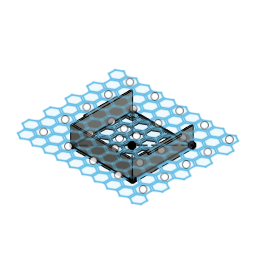
SC846-rear-fan-80mm v2 (Autodesk Fusion 360 design; units mm, degrees)
Autodesk Fusion 360 part; units mm, degrees
sketch "Sketch1" plane through (0, 0, 0) normal (0, 1, 0) x (1, 0, 0)
  line L0 (42.25, -41.5) -> (-42.25, -41.5)
  line L1 (-42.25, -41.5) -> (-42.25, 41.5)
  line L2 (-42.25, 41.5) -> (42.25, 41.5)
  line L3 (42.25, 41.5) -> (42.25, -41.5)
  line L4 (42.25, -41.5) -> (-42.25, 41.5) construction
  line L5 (-42.25, -41.5) -> (42.25, 41.5) construction
  dimension "d1" = 84.5
  dimension "d2" = 83
  constraint horizontal L0
  constraint perpendicular L0 L1
  constraint parallel L0 L2
  constraint parallel L1 L3
  constraint coincident L4 origin
  constraint coincident L5 origin
  measures "d1" distance of L0.start L0.end
  measures "d2" distance of L0.start L2.end
extrude "Extrude1" add sketch "Sketch1" along normal blind 3
sketch "Sketch2" plane through (0, 3, 0) normal (0, 1, 0) x (-1, 0, 0)
  line L0 (-42.25, -41.5) -> (42.25, -41.5)
  line L1 (42.25, -41.5) -> (42.25, 41.5)
  line L2 (42.25, 41.5) -> (-42.25, 41.5)
  line L3 (-42.25, 41.5) -> (-42.25, -41.5)
  line L4 (42.25, 41.5) -> (-42.25, 41.5)
  line L5 (-42.25, 41.5) -> (-42.25, 39.5)
  line L6 (-42.25, 39.5) -> (42.25, 39.5)
  line L7 (42.25, 39.5) -> (42.25, 41.5)
  dimension "d5" = 2
  constraint horizontal L4
  constraint vertical L5
  constraint horizontal L6
  constraint vertical L7
  constraint coincident L3 L5.end
  constraint coincident L1.end L2.start
  measures "d5" distance of L2.end L5.end
extrude "Extrude2" add sketch "Sketch2" along normal blind 24.5 contours L1 L2 L3 L4 L5 L6 L7
sketch "Sketch3" plane through (0, 0, 0) normal (0, 1, 0) x (1, 0, 0)
  line L0 (42.25, 41.5, 3) -> (40.5, 41.5, 3)
  line L1 (40.5, 41.5, 3) -> (40.5, -39.5, 3)
  line L2 (40.5, -39.5, 3) -> (42.25, -39.5, 3)
  line L3 (42.25, -39.5, 3) -> (42.25, 41.5, 3)
  line L4 (-42.25, -39.5, 3) -> (42.25, -39.5, 3)
  point P0 (42.25, 41.5)
  dimension "d8" = 1.75
extrude "Extrude3" add sketch "Sketch3" along normal up to surface (24.5 mm away) contours L0 L1 L2 L3 L4 in plane through (0, 3, 0) normal (0, 1, 0)
sketch "Sketch4" plane through (0, 3, 0) normal (0, 1, 0) x (-1, 0, 0)
  line L0 (-40.5, 39.5) -> (-40.5, -41.5)
  line L1 (-40.5, -41.5) -> (42.25, -41.5)
  line L2 (42.25, -41.5) -> (42.25, 39.5)
  line L3 (42.25, 39.5) -> (-40.5, 39.5)
  line L4 (42.25, 39.5) -> (40.5, 39.5)
  line L5 (40.5, 39.5) -> (40.5, -41.5)
  line L6 (40.5, -41.5) -> (42.25, -41.5)
  line L7 (42.25, -41.5) -> (42.25, 39.5)
  dimension "d11" = 1.75
  constraint horizontal L4
  constraint vertical L5
  constraint horizontal L6
  constraint vertical L7
  constraint coincident L1 L5.end
  constraint coincident L2.end L3.start
  measures "d11" distance of L5.end L1.end
extrude "Extrude4" add sketch "Sketch4" along normal up to surface (24.5 mm away) contours L1 L2 L3 L4 L5 L6 L7
sketch "Sketch5" plane through (0, 3, 0) normal (0, 1, 0) x (-1, 0, 0)
  line L0 (40.5, -41.5) -> (40.5, 39.5)
  line L1 (40.5, 39.5) -> (-40.5, 39.5)
  line L2 (-40.5, 39.5) -> (-40.5, -41.5)
  line L3 (-40.5, -41.5) -> (40.5, -41.5)
  line L4 (-40.5, -41.5) -> (40.5, 39.5) construction
  line L5 (40.5, -41.5) -> (-40.5, 39.5) construction
  constraint coincident L2.end L3.start
  constraint coincident L0.end L1.start
  constraint coincident L0.start L3.end
  constraint coincident L1.end L2.start
sketch "Sketch11" plane through (42.25, 0, 0) normal (1, 0, 0) x (0, 0, -1)
  line L0 (-41.5, 0) -> (41.5, 0)
  line L1 (41.5, 0) -> (41.5, 27.5)
  line L2 (41.5, 27.5) -> (-41.5, 27.5)
  line L3 (-41.5, 27.5) -> (-41.5, 0)
  line L4 (-21.5, 27.5) -> (23.5, 27.5)
  line L5 (23.5, 27.5) -> (23.5, 25)
  line L6 (23.5, 25) -> (-21.5, 25)
  line L7 (-21.5, 25) -> (-21.5, 27.5)
  dimension "d58" = 2.5
  dimension "d59" = 20
  dimension "d60" = 45
  constraint horizontal L4
  constraint vertical L5
  constraint horizontal L6
  constraint vertical L7
  constraint coincident L2 L4.start
  measures "d58" distance of L4.start L6.end
  measures "d59" distance of L3 L7
  measures "d60" distance of L5.end L6.end
extrude "Extrude6" add sketch "Sketch11" along normal blind 2 contours L2 L4 L5 L6 L7
sketch "Sketch12" plane through (-42.25, 0, 0) normal (-1, 0, 0) x (0, 0, 1)
  line L0 (-41.5, 0) -> (41.5, 0)
  line L1 (41.5, 0) -> (41.5, 27.5)
  line L2 (41.5, 27.5) -> (-41.5, 27.5)
  line L3 (-41.5, 27.5) -> (-41.5, 0)
  line L4 (21.5, 27.5) -> (-23.5, 27.5)
  line L5 (-23.5, 27.5) -> (-23.5, 25)
  line L6 (-23.5, 25) -> (21.5, 25)
  line L7 (21.5, 25) -> (21.5, 27.5)
  dimension "d63" = 2.5
  dimension "d64" = 45
  dimension "d65" = 20
  constraint horizontal L4
  constraint vertical L5
  constraint horizontal L6
  constraint vertical L7
  constraint coincident L2 L4.start
  measures "d63" distance of L4.start L6.end
  measures "d64" distance of L5.end L6.end
  measures "d65" distance of L1.end L4.start
extrude "Extrude7" add sketch "Sketch12" along normal blind 2 contours L2 L4 L5 L6 L7
sketch "Sketch13" plane through (0, 3, -1) normal (0, 1, 0) x (-1, 0, 0)
  line L0 (40.5, 40.5) -> (31, 40.5)
  line L1 (31, 40.5) -> (31, 31)
  line L2 (31, 31) -> (40.5, 31)
  line L3 (40.5, 31) -> (40.5, 40.5)
  line L4 (-40.5, -40.5) -> (40.5, 40.5)
  line L5 (40.5, -40.5) -> (31, -40.5)
  line L6 (31, -40.5) -> (31, -31)
  line L7 (31, -31) -> (40.5, -31)
  line L8 (40.5, -31) -> (40.5, -40.5)
  line L9 (40.5, -40.5) -> (-40.5, 40.5)
  line L10 (-40.5, 40.5) -> (-31, 40.5)
  line L11 (-31, 40.5) -> (-31, 31)
  line L12 (-31, 31) -> (-40.5, 31)
  line L13 (-40.5, 31) -> (-40.5, 40.5)
  line L14 (-40.5, -40.5) -> (-31, -40.5)
  line L15 (-31, -40.5) -> (-31, -31)
  line L16 (-31, -31) -> (-40.5, -31)
  line L17 (-40.5, -31) -> (-40.5, -40.5)
  line L18 (40.5, 40.5) -> (-40.5, 40.5)
  line L19 (-40.5, 40.5) -> (-40.5, -40.5)
  line L20 (-40.5, -40.5) -> (40.5, -40.5)
  line L21 (40.5, -40.5) -> (40.5, 40.5)
  line L22 (40.5, 40.5) -> (-40.5, -40.5) construction
  line L23 (-40.5, 40.5) -> (40.5, -40.5) construction
  point P0 (40.5, 40.5)
  point P1 (40.5, -40.5)
  constraint horizontal L0
  constraint vertical L1
  constraint horizontal L2
  constraint vertical L3
  constraint coincident L1.end L4
  constraint coincident P0 L0.start
  constraint horizontal L5
  constraint vertical L6
  constraint horizontal L7
  constraint vertical L8
  constraint coincident L6.end L9
  constraint coincident P1 L5.start
  constraint horizontal L10
  constraint vertical L11
  constraint horizontal L12
  constraint vertical L13
  constraint coincident L9 L11.end
  constraint coincident L9.end L10.start
  constraint horizontal L14
  constraint vertical L15
  constraint horizontal L16
  constraint vertical L17
  constraint coincident L4 L15.end
  constraint coincident L4.start L14.start
  constraint horizontal L18
  constraint perpendicular L18 L19
  constraint parallel L18 L20
  constraint parallel L19 L21
  constraint coincident L22 origin
  constraint coincident L23 origin
extrude "Extrude8" cut sketch "Sketch13" against normal through all contours L1 L4 L9 L11 L18 | L2 L4 L7 L9 L21 | L4 L6 L9 L15 L20 | L4 L9 L12 L16 L19
fillet "Fillet3" radius 4.5 4 edges at (31, 1.5, 30) (-31, 1.5, -32) (-31, 1.5, 30) (31, 1.5, -32)
sketch "Sketch15" plane through (0, 0, -41.5) normal (0, 0, -1) x (-1, 0, 0)
  line L0 (-31, 0) -> (-31, 3)
  line L1 (-31, 3) -> (-40.5, 3)
  line L2 (-40.5, 3) -> (-40.5, 27.5)
  line L3 (-40.5, 27.5) -> (-42.25, 27.5)
  line L4 (-42.25, 27.5) -> (-42.25, 0)
  line L5 (-42.25, 0) -> (-31, 0)
  line L6 (-42.25, 0) -> (42.25, 0)
  line L7 (42.25, 0) -> (42.25, 3)
  line L8 (42.25, 3) -> (-42.25, 3)
  line L9 (-42.25, 3) -> (-42.25, 0)
  line L10 (42.25, 0) -> (42.25, 27.5)
  constraint horizontal L6
  constraint vertical L7
  constraint horizontal L8
  constraint vertical L9
  constraint coincident L7.end L10
  constraint coincident L4.end L5.start
extrude "Extrude9" add sketch "Sketch15" along normal blind 2 contours L0 L1 L4 L5 L6 L8 L9 | L0 L6 L7 L8 L10
sketch "Sketch16" plane through (0, 27.5, 0) normal (0, 1, 0) x (-1, 0, 0)
  line L0 (42.25, 21.5) -> (42.25, 41.5)
  line L1 (42.25, 41.5) -> (-42.25, 41.5)
  line L2 (-42.25, 41.5) -> (-42.25, 21.5)
  line L3 (-42.25, 21.5) -> (-44.25, 21.5)
  line L4 (-44.25, 21.5) -> (-44.25, -23.5)
  line L5 (-44.25, -23.5) -> (-42.25, -23.5)
  line L6 (-42.25, -23.5) -> (-42.25, -41.5)
  line L7 (-42.25, -41.5) -> (-40.5, -41.5)
  line L8 (-40.5, -41.5) -> (-40.5, 39.5)
  line L9 (-40.5, 39.5) -> (40.5, 39.5)
  line L10 (40.5, 39.5) -> (40.5, -41.5)
  line L11 (40.5, -41.5) -> (42.25, -41.5)
  line L12 (42.25, -41.5) -> (42.25, -23.5)
  line L13 (42.25, -23.5) -> (44.25, -23.5)
  line L14 (44.25, -23.5) -> (44.25, 21.5)
  line L15 (44.25, 21.5) -> (42.25, 21.5)
  line L16 (-25.5, 39.5) -> (-20.5, 39.5)
  line L17 (-20.5, 39.5) -> (-20.5, 41.5)
  line L18 (-20.5, 41.5) -> (-25.5, 41.5)
  line L19 (-25.5, 41.5) -> (-25.5, 39.5)
  dimension "d73" = 15
  dimension "d74" = 5
  constraint horizontal L16
  constraint vertical L17
  constraint horizontal L18
  constraint vertical L19
  constraint coincident L1 L17.end
  constraint coincident L9 L16.start
  measures "d73" distance of L8.end L16.start
  measures "d74" distance of L16.start L16.end
extrude "Extrude10" cut sketch "Sketch16" against normal blind 5 contours L1 L9 L16 L17 L18 L19
fillet "Fillet4" radius 1 4 edges at (25.5, 22.5, 40.5) (25.5, 27.5, 40.5) (20.5, 22.5, 40.5) (20.5, 27.5, 40.5)
fillet "Fillet5" radius 1 2 edges at (0, 3, -43.5) (0, 0, -43.5)
sketch "Sketch17" plane through (0, 3, 0) normal (0, 1, 0) x (-1, 0, 0)
  line L0 (-7.5, -4.3301) -> (0, -8.6603)
  line L1 (0, -8.6603) -> (7.5, -4.3301)
  line L2 (7.5, -4.3301) -> (7.5, 4.3301)
  line L3 (7.5, 4.3301) -> (0, 8.6603)
  line L4 (0, 8.6603) -> (-7.5, 4.3301)
  line L5 (-7.5, 4.3301) -> (-7.5, -4.3301)
  line L6 (9.5, -4.3301) -> (17, -8.6603)
  line L7 (17, -8.6603) -> (24.5, -4.3301)
  line L8 (24.5, -4.3301) -> (24.5, 4.3301)
  line L9 (24.5, 4.3301) -> (17, 8.6603)
  line L10 (17, 8.6603) -> (9.5, 4.3301)
  line L11 (9.5, 4.3301) -> (9.5, -4.3301)
  line L12 (1, -19.0526) -> (8.5, -23.3827)
  line L13 (8.5, -23.3827) -> (16, -19.0526)
  line L14 (16, -19.0526) -> (16, -10.3923)
  line L15 (16, -10.3923) -> (8.5, -6.0622)
  line L16 (8.5, -6.0622) -> (1, -10.3923)
  line L17 (1, -10.3923) -> (1, -19.0526)
  line L18 (18, -19.0526) -> (25.5, -23.3827)
  line L19 (25.5, -23.3827) -> (33, -19.0526)
  line L20 (33, -19.0526) -> (33, -10.3923)
  line L21 (33, -10.3923) -> (25.5, -6.0622)
  line L22 (25.5, -6.0622) -> (18, -10.3923)
  line L23 (18, -10.3923) -> (18, -19.0526)
  line L24 (-42.5, -82.3827) -> (-35, -78.0526)
  line L25 (-50, -69.3923) -> (-50, -78.0526)
  line L26 (-52, -69.3923) -> (-59.5, -65.0622)
  line L27 (-60.5, -63.3301) -> (-60.5, -54.6699)
  line L28 (-68, -67.6603) -> (-60.5, -63.3301)
  line L29 (-59.5, -65.0622) -> (-67, -69.3923)
  line L30 (-52, -78.0526) -> (-52, -69.3923)
  line L31 (-59.5, -82.3827) -> (-52, -78.0526)
  line L32 (-67, -78.0526) -> (-59.5, -82.3827)
  line L33 (-67, -69.3923) -> (-67, -78.0526)
  line L34 (-75.5, -63.3301) -> (-68, -67.6603)
  line L35 (-58.5, -63.3301) -> (-51, -67.6603)
  line L36 (-58.5, -54.6699) -> (-58.5, -63.3301)
  line L37 (-60.5, -54.6699) -> (-68, -50.3397)
  line L38 (-68, -50.3397) -> (-75.5, -54.6699)
  line L39 (-75.5, -54.6699) -> (-75.5, -63.3301)
  line L40 (-51, -50.3397) -> (-58.5, -54.6699)
  line L41 (-43.5, -54.6699) -> (-51, -50.3397)
  line L42 (-43.5, -63.3301) -> (-43.5, -54.6699)
  line L43 (-51, -67.6603) -> (-43.5, -63.3301)
  line L44 (-42.5, -65.0622) -> (-50, -69.3923)
  line L45 (-50, -78.0526) -> (-42.5, -82.3827)
  line L46 (-35, -78.0526) -> (-35, -69.3923)
  line L47 (-35, -69.3923) -> (-42.5, -65.0622)
  line L48 (-8.5, -82.3827) -> (-1, -78.0526)
  line L49 (-16, -69.3923) -> (-16, -78.0526)
  line L50 (-18, -69.3923) -> (-25.5, -65.0622)
  line L51 (-26.5, -63.3301) -> (-26.5, -54.6699)
  line L52 (-34, -67.6603) -> (-26.5, -63.3301)
  line L53 (-25.5, -65.0622) -> (-33, -69.3923)
  line L54 (-18, -78.0526) -> (-18, -69.3923)
  line L55 (-25.5, -82.3827) -> (-18, -78.0526)
  line L56 (-33, -78.0526) -> (-25.5, -82.3827)
  line L57 (-33, -69.3923) -> (-33, -78.0526)
  line L58 (-41.5, -63.3301) -> (-34, -67.6603)
  line L59 (-24.5, -63.3301) -> (-17, -67.6603)
  line L60 (-24.5, -54.6699) -> (-24.5, -63.3301)
  line L61 (-26.5, -54.6699) -> (-34, -50.3397)
  line L62 (-34, -50.3397) -> (-41.5, -54.6699)
  line L63 (-41.5, -54.6699) -> (-41.5, -63.3301)
  line L64 (-17, -50.3397) -> (-24.5, -54.6699)
  line L65 (-9.5, -54.6699) -> (-17, -50.3397)
  line L66 (-9.5, -63.3301) -> (-9.5, -54.6699)
  line L67 (-17, -67.6603) -> (-9.5, -63.3301)
  line L68 (-8.5, -65.0622) -> (-16, -69.3923)
  line L69 (-16, -78.0526) -> (-8.5, -82.3827)
  line L70 (-1, -78.0526) -> (-1, -69.3923)
  line L71 (-1, -69.3923) -> (-8.5, -65.0622)
  line L72 (25.5, -82.3827) -> (33, -78.0526)
  line L73 (18, -69.3923) -> (18, -78.0526)
  line L74 (16, -69.3923) -> (8.5, -65.0622)
  line L75 (7.5, -63.3301) -> (7.5, -54.6699)
  line L76 (0, -67.6603) -> (7.5, -63.3301)
  line L77 (8.5, -65.0622) -> (1, -69.3923)
  line L78 (16, -78.0526) -> (16, -69.3923)
  line L79 (8.5, -82.3827) -> (16, -78.0526)
  line L80 (1, -78.0526) -> (8.5, -82.3827)
  line L81 (1, -69.3923) -> (1, -78.0526)
  line L82 (-7.5, -63.3301) -> (0, -67.6603)
  line L83 (9.5, -63.3301) -> (17, -67.6603)
  line L84 (9.5, -54.6699) -> (9.5, -63.3301)
  line L85 (7.5, -54.6699) -> (0, -50.3397)
  line L86 (0, -50.3397) -> (-7.5, -54.6699)
  line L87 (-7.5, -54.6699) -> (-7.5, -63.3301)
  line L88 (17, -50.3397) -> (9.5, -54.6699)
  line L89 (24.5, -54.6699) -> (17, -50.3397)
  line L90 (24.5, -63.3301) -> (24.5, -54.6699)
  line L91 (17, -67.6603) -> (24.5, -63.3301)
  line L92 (25.5, -65.0622) -> (18, -69.3923)
  line L93 (18, -78.0526) -> (25.5, -82.3827)
  line L94 (33, -78.0526) -> (33, -69.3923)
  line L95 (33, -69.3923) -> (25.5, -65.0622)
  line L96 (59.5, -82.3827) -> (67, -78.0526)
  line L97 (52, -69.3923) -> (52, -78.0526)
  line L98 (50, -69.3923) -> (42.5, -65.0622)
  line L99 (41.5, -63.3301) -> (41.5, -54.6699)
  line L100 (34, -67.6603) -> (41.5, -63.3301)
  line L101 (42.5, -65.0622) -> (35, -69.3923)
  line L102 (50, -78.0526) -> (50, -69.3923)
  line L103 (42.5, -82.3827) -> (50, -78.0526)
  line L104 (35, -78.0526) -> (42.5, -82.3827)
  line L105 (35, -69.3923) -> (35, -78.0526)
  line L106 (26.5, -63.3301) -> (34, -67.6603)
  line L107 (43.5, -63.3301) -> (51, -67.6603)
  line L108 (43.5, -54.6699) -> (43.5, -63.3301)
  line L109 (41.5, -54.6699) -> (34, -50.3397)
  line L110 (34, -50.3397) -> (26.5, -54.6699)
  line L111 (26.5, -54.6699) -> (26.5, -63.3301)
  line L112 (51, -50.3397) -> (43.5, -54.6699)
  line L113 (58.5, -54.6699) -> (51, -50.3397)
  line L114 (58.5, -63.3301) -> (58.5, -54.6699)
  line L115 (51, -67.6603) -> (58.5, -63.3301)
  line L116 (59.5, -65.0622) -> (52, -69.3923)
  line L117 (52, -78.0526) -> (59.5, -82.3827)
  line L118 (67, -78.0526) -> (67, -69.3923)
  line L119 (67, -69.3923) -> (59.5, -65.0622)
  line L120 (93.5, -82.3827) -> (101, -78.0526)
  line L121 (86, -69.3923) -> (86, -78.0526)
  line L122 (84, -69.3923) -> (76.5, -65.0622)
  line L123 (75.5, -63.3301) -> (75.5, -54.6699)
  line L124 (68, -67.6603) -> (75.5, -63.3301)
  line L125 (76.5, -65.0622) -> (69, -69.3923)
  line L126 (84, -78.0526) -> (84, -69.3923)
  line L127 (76.5, -82.3827) -> (84, -78.0526)
  line L128 (69, -78.0526) -> (76.5, -82.3827)
  line L129 (69, -69.3923) -> (69, -78.0526)
  line L130 (60.5, -63.3301) -> (68, -67.6603)
  line L131 (77.5, -63.3301) -> (85, -67.6603)
  line L132 (77.5, -54.6699) -> (77.5, -63.3301)
  line L133 (75.5, -54.6699) -> (68, -50.3397)
  line L134 (68, -50.3397) -> (60.5, -54.6699)
  line L135 (60.5, -54.6699) -> (60.5, -63.3301)
  line L136 (85, -50.3397) -> (77.5, -54.6699)
  line L137 (92.5, -54.6699) -> (85, -50.3397)
  line L138 (92.5, -63.3301) -> (92.5, -54.6699)
  line L139 (85, -67.6603) -> (92.5, -63.3301)
  line L140 (93.5, -65.0622) -> (86, -69.3923)
  line L141 (86, -78.0526) -> (93.5, -82.3827)
  line L142 (101, -78.0526) -> (101, -69.3923)
  line L143 (101, -69.3923) -> (93.5, -65.0622)
  line L144 (-42.5, -52.8827) -> (-35, -48.5526)
  line L145 (-50, -39.8923) -> (-50, -48.5526)
  line L146 (-52, -39.8923) -> (-59.5, -35.5622)
  line L147 (-60.5, -33.8301) -> (-60.5, -25.1699)
  line L148 (-68, -38.1603) -> (-60.5, -33.8301)
  line L149 (-59.5, -35.5622) -> (-67, -39.8923)
  line L150 (-52, -48.5526) -> (-52, -39.8923)
  line L151 (-59.5, -52.8827) -> (-52, -48.5526)
  line L152 (-67, -48.5526) -> (-59.5, -52.8827)
  line L153 (-67, -39.8923) -> (-67, -48.5526)
  line L154 (-75.5, -33.8301) -> (-68, -38.1603)
  line L155 (-58.5, -33.8301) -> (-51, -38.1603)
  line L156 (-58.5, -25.1699) -> (-58.5, -33.8301)
  line L157 (-60.5, -25.1699) -> (-68, -20.8397)
  line L158 (-68, -20.8397) -> (-75.5, -25.1699)
  line L159 (-75.5, -25.1699) -> (-75.5, -33.8301)
  line L160 (-51, -20.8397) -> (-58.5, -25.1699)
  line L161 (-43.5, -25.1699) -> (-51, -20.8397)
  line L162 (-43.5, -33.8301) -> (-43.5, -25.1699)
  line L163 (-51, -38.1603) -> (-43.5, -33.8301)
  line L164 (-42.5, -35.5622) -> (-50, -39.8923)
  line L165 (-50, -48.5526) -> (-42.5, -52.8827)
  line L166 (-35, -48.5526) -> (-35, -39.8923)
  line L167 (-35, -39.8923) -> (-42.5, -35.5622)
  line L168 (-8.5, -52.8827) -> (-1, -48.5526)
  line L169 (-16, -39.8923) -> (-16, -48.5526)
  line L170 (-18, -39.8923) -> (-25.5, -35.5622)
  line L171 (-26.5, -33.8301) -> (-26.5, -25.1699)
  line L172 (-34, -38.1603) -> (-26.5, -33.8301)
  line L173 (-25.5, -35.5622) -> (-33, -39.8923)
  line L174 (-18, -48.5526) -> (-18, -39.8923)
  line L175 (-25.5, -52.8827) -> (-18, -48.5526)
  line L176 (-33, -48.5526) -> (-25.5, -52.8827)
  line L177 (-33, -39.8923) -> (-33, -48.5526)
  line L178 (-41.5, -33.8301) -> (-34, -38.1603)
  line L179 (-24.5, -33.8301) -> (-17, -38.1603)
  line L180 (-24.5, -25.1699) -> (-24.5, -33.8301)
  line L181 (-26.5, -25.1699) -> (-34, -20.8397)
  line L182 (-34, -20.8397) -> (-41.5, -25.1699)
  line L183 (-41.5, -25.1699) -> (-41.5, -33.8301)
  line L184 (-17, -20.8397) -> (-24.5, -25.1699)
  line L185 (-9.5, -25.1699) -> (-17, -20.8397)
  line L186 (-9.5, -33.8301) -> (-9.5, -25.1699)
  line L187 (-17, -38.1603) -> (-9.5, -33.8301)
  line L188 (-8.5, -35.5622) -> (-16, -39.8923)
  line L189 (-16, -48.5526) -> (-8.5, -52.8827)
  line L190 (-1, -48.5526) -> (-1, -39.8923)
  line L191 (-1, -39.8923) -> (-8.5, -35.5622)
  line L192 (25.5, -52.8827) -> (33, -48.5526)
  line L193 (18, -39.8923) -> (18, -48.5526)
  line L194 (16, -39.8923) -> (8.5, -35.5622)
  line L195 (7.5, -33.8301) -> (7.5, -25.1699)
  line L196 (0, -38.1603) -> (7.5, -33.8301)
  line L197 (8.5, -35.5622) -> (1, -39.8923)
  line L198 (16, -48.5526) -> (16, -39.8923)
  line L199 (8.5, -52.8827) -> (16, -48.5526)
  line L200 (1, -48.5526) -> (8.5, -52.8827)
  line L201 (1, -39.8923) -> (1, -48.5526)
  line L202 (-7.5, -33.8301) -> (0, -38.1603)
  line L203 (9.5, -33.8301) -> (17, -38.1603)
  line L204 (9.5, -25.1699) -> (9.5, -33.8301)
  line L205 (7.5, -25.1699) -> (0, -20.8397)
  line L206 (0, -20.8397) -> (-7.5, -25.1699)
  line L207 (-7.5, -25.1699) -> (-7.5, -33.8301)
  line L208 (17, -20.8397) -> (9.5, -25.1699)
  line L209 (24.5, -25.1699) -> (17, -20.8397)
  line L210 (24.5, -33.8301) -> (24.5, -25.1699)
  line L211 (17, -38.1603) -> (24.5, -33.8301)
  line L212 (25.5, -35.5622) -> (18, -39.8923)
  line L213 (18, -48.5526) -> (25.5, -52.8827)
  line L214 (33, -48.5526) -> (33, -39.8923)
  line L215 (33, -39.8923) -> (25.5, -35.5622)
  line L216 (59.5, -52.8827) -> (67, -48.5526)
  line L217 (52, -39.8923) -> (52, -48.5526)
  line L218 (50, -39.8923) -> (42.5, -35.5622)
  line L219 (41.5, -33.8301) -> (41.5, -25.1699)
  line L220 (34, -38.1603) -> (41.5, -33.8301)
  line L221 (42.5, -35.5622) -> (35, -39.8923)
  line L222 (50, -48.5526) -> (50, -39.8923)
  line L223 (42.5, -52.8827) -> (50, -48.5526)
  line L224 (35, -48.5526) -> (42.5, -52.8827)
  line L225 (35, -39.8923) -> (35, -48.5526)
  line L226 (26.5, -33.8301) -> (34, -38.1603)
  line L227 (43.5, -33.8301) -> (51, -38.1603)
  line L228 (43.5, -25.1699) -> (43.5, -33.8301)
  line L229 (41.5, -25.1699) -> (34, -20.8397)
  line L230 (34, -20.8397) -> (26.5, -25.1699)
  line L231 (26.5, -25.1699) -> (26.5, -33.8301)
  line L232 (51, -20.8397) -> (43.5, -25.1699)
  line L233 (58.5, -25.1699) -> (51, -20.8397)
  line L234 (58.5, -33.8301) -> (58.5, -25.1699)
  line L235 (51, -38.1603) -> (58.5, -33.8301)
  line L236 (59.5, -35.5622) -> (52, -39.8923)
  line L237 (52, -48.5526) -> (59.5, -52.8827)
  line L238 (67, -48.5526) -> (67, -39.8923)
  line L239 (67, -39.8923) -> (59.5, -35.5622)
  line L240 (93.5, -52.8827) -> (101, -48.5526)
  line L241 (86, -39.8923) -> (86, -48.5526)
  line L242 (84, -39.8923) -> (76.5, -35.5622)
  line L243 (75.5, -33.8301) -> (75.5, -25.1699)
  line L244 (68, -38.1603) -> (75.5, -33.8301)
  line L245 (76.5, -35.5622) -> (69, -39.8923)
  line L246 (84, -48.5526) -> (84, -39.8923)
  line L247 (76.5, -52.8827) -> (84, -48.5526)
  line L248 (69, -48.5526) -> (76.5, -52.8827)
  line L249 (69, -39.8923) -> (69, -48.5526)
  line L250 (60.5, -33.8301) -> (68, -38.1603)
  line L251 (77.5, -33.8301) -> (85, -38.1603)
  line L252 (77.5, -25.1699) -> (77.5, -33.8301)
  line L253 (75.5, -25.1699) -> (68, -20.8397)
  line L254 (68, -20.8397) -> (60.5, -25.1699)
  line L255 (60.5, -25.1699) -> (60.5, -33.8301)
  line L256 (85, -20.8397) -> (77.5, -25.1699)
  line L257 (92.5, -25.1699) -> (85, -20.8397)
  line L258 (92.5, -33.8301) -> (92.5, -25.1699)
  line L259 (85, -38.1603) -> (92.5, -33.8301)
  line L260 (93.5, -35.5622) -> (86, -39.8923)
  line L261 (86, -48.5526) -> (93.5, -52.8827)
  line L262 (101, -48.5526) -> (101, -39.8923)
  line L263 (101, -39.8923) -> (93.5, -35.5622)
  line L264 (-42.5, -23.3827) -> (-35, -19.0526)
  line L265 (-50, -10.3923) -> (-50, -19.0526)
  line L266 (-52, -10.3923) -> (-59.5, -6.0622)
  line L267 (-60.5, -4.3301) -> (-60.5, 4.3301)
  line L268 (-68, -8.6603) -> (-60.5, -4.3301)
  line L269 (-59.5, -6.0622) -> (-67, -10.3923)
  line L270 (-52, -19.0526) -> (-52, -10.3923)
  line L271 (-59.5, -23.3827) -> (-52, -19.0526)
  line L272 (-67, -19.0526) -> (-59.5, -23.3827)
  line L273 (-67, -10.3923) -> (-67, -19.0526)
  line L274 (-75.5, -4.3301) -> (-68, -8.6603)
  line L275 (-58.5, -4.3301) -> (-51, -8.6603)
  line L276 (-58.5, 4.3301) -> (-58.5, -4.3301)
  line L277 (-60.5, 4.3301) -> (-68, 8.6603)
  line L278 (-68, 8.6603) -> (-75.5, 4.3301)
  line L279 (-75.5, 4.3301) -> (-75.5, -4.3301)
  line L280 (-51, 8.6603) -> (-58.5, 4.3301)
  line L281 (-43.5, 4.3301) -> (-51, 8.6603)
  line L282 (-43.5, -4.3301) -> (-43.5, 4.3301)
  line L283 (-51, -8.6603) -> (-43.5, -4.3301)
  line L284 (-42.5, -6.0622) -> (-50, -10.3923)
  line L285 (-50, -19.0526) -> (-42.5, -23.3827)
  line L286 (-35, -19.0526) -> (-35, -10.3923)
  line L287 (-35, -10.3923) -> (-42.5, -6.0622)
  line L288 (-8.5, -23.3827) -> (-1, -19.0526)
  line L289 (-16, -10.3923) -> (-16, -19.0526)
  line L290 (-18, -10.3923) -> (-25.5, -6.0622)
  line L291 (-26.5, -4.3301) -> (-26.5, 4.3301)
  line L292 (-34, -8.6603) -> (-26.5, -4.3301)
  line L293 (-25.5, -6.0622) -> (-33, -10.3923)
  line L294 (-18, -19.0526) -> (-18, -10.3923)
  line L295 (-25.5, -23.3827) -> (-18, -19.0526)
  line L296 (-33, -19.0526) -> (-25.5, -23.3827)
  line L297 (-33, -10.3923) -> (-33, -19.0526)
  line L298 (-41.5, -4.3301) -> (-34, -8.6603)
  line L299 (-24.5, -4.3301) -> (-17, -8.6603)
  line L300 (-24.5, 4.3301) -> (-24.5, -4.3301)
  line L301 (-26.5, 4.3301) -> (-34, 8.6603)
  line L302 (-34, 8.6603) -> (-41.5, 4.3301)
  line L303 (-41.5, 4.3301) -> (-41.5, -4.3301)
  line L304 (-17, 8.6603) -> (-24.5, 4.3301)
  line L305 (-9.5, 4.3301) -> (-17, 8.6603)
  line L306 (-9.5, -4.3301) -> (-9.5, 4.3301)
  line L307 (-17, -8.6603) -> (-9.5, -4.3301)
  line L308 (-8.5, -6.0622) -> (-16, -10.3923)
  line L309 (-16, -19.0526) -> (-8.5, -23.3827)
  line L310 (-1, -19.0526) -> (-1, -10.3923)
  line L311 (-1, -10.3923) -> (-8.5, -6.0622)
  line L312 (59.5, -23.3827) -> (67, -19.0526)
  line L313 (52, -10.3923) -> (52, -19.0526)
  line L314 (50, -10.3923) -> (42.5, -6.0622)
  line L315 (41.5, -4.3301) -> (41.5, 4.3301)
  line L316 (34, -8.6603) -> (41.5, -4.3301)
  line L317 (42.5, -6.0622) -> (35, -10.3923)
  line L318 (50, -19.0526) -> (50, -10.3923)
  line L319 (42.5, -23.3827) -> (50, -19.0526)
  line L320 (35, -19.0526) -> (42.5, -23.3827)
  line L321 (35, -10.3923) -> (35, -19.0526)
  line L322 (26.5, -4.3301) -> (34, -8.6603)
  line L323 (43.5, -4.3301) -> (51, -8.6603)
  line L324 (43.5, 4.3301) -> (43.5, -4.3301)
  line L325 (41.5, 4.3301) -> (34, 8.6603)
  line L326 (34, 8.6603) -> (26.5, 4.3301)
  line L327 (26.5, 4.3301) -> (26.5, -4.3301)
  line L328 (51, 8.6603) -> (43.5, 4.3301)
  line L329 (58.5, 4.3301) -> (51, 8.6603)
  line L330 (58.5, -4.3301) -> (58.5, 4.3301)
  line L331 (51, -8.6603) -> (58.5, -4.3301)
  line L332 (59.5, -6.0622) -> (52, -10.3923)
  line L333 (52, -19.0526) -> (59.5, -23.3827)
  line L334 (67, -19.0526) -> (67, -10.3923)
  line L335 (67, -10.3923) -> (59.5, -6.0622)
  line L336 (93.5, -23.3827) -> (101, -19.0526)
  line L337 (86, -10.3923) -> (86, -19.0526)
  line L338 (84, -10.3923) -> (76.5, -6.0622)
  line L339 (75.5, -4.3301) -> (75.5, 4.3301)
  line L340 (68, -8.6603) -> (75.5, -4.3301)
  line L341 (76.5, -6.0622) -> (69, -10.3923)
  line L342 (84, -19.0526) -> (84, -10.3923)
  line L343 (76.5, -23.3827) -> (84, -19.0526)
  line L344 (69, -19.0526) -> (76.5, -23.3827)
  line L345 (69, -10.3923) -> (69, -19.0526)
  line L346 (60.5, -4.3301) -> (68, -8.6603)
  line L347 (77.5, -4.3301) -> (85, -8.6603)
  line L348 (77.5, 4.3301) -> (77.5, -4.3301)
  line L349 (75.5, 4.3301) -> (68, 8.6603)
  line L350 (68, 8.6603) -> (60.5, 4.3301)
  line L351 (60.5, 4.3301) -> (60.5, -4.3301)
  line L352 (85, 8.6603) -> (77.5, 4.3301)
  line L353 (92.5, 4.3301) -> (85, 8.6603)
  line L354 (92.5, -4.3301) -> (92.5, 4.3301)
  line L355 (85, -8.6603) -> (92.5, -4.3301)
  line L356 (93.5, -6.0622) -> (86, -10.3923)
  line L357 (86, -19.0526) -> (93.5, -23.3827)
  line L358 (101, -19.0526) -> (101, -10.3923)
  line L359 (101, -10.3923) -> (93.5, -6.0622)
  line L360 (-42.5, 6.1173) -> (-35, 10.4474)
  line L361 (-50, 19.1077) -> (-50, 10.4474)
  line L362 (-52, 19.1077) -> (-59.5, 23.4378)
  line L363 (-60.5, 25.1699) -> (-60.5, 33.8301)
  line L364 (-68, 20.8397) -> (-60.5, 25.1699)
  line L365 (-59.5, 23.4378) -> (-67, 19.1077)
  line L366 (-52, 10.4474) -> (-52, 19.1077)
  line L367 (-59.5, 6.1173) -> (-52, 10.4474)
  line L368 (-67, 10.4474) -> (-59.5, 6.1173)
  line L369 (-67, 19.1077) -> (-67, 10.4474)
  line L370 (-75.5, 25.1699) -> (-68, 20.8397)
  line L371 (-58.5, 25.1699) -> (-51, 20.8397)
  line L372 (-58.5, 33.8301) -> (-58.5, 25.1699)
  line L373 (-60.5, 33.8301) -> (-68, 38.1603)
  line L374 (-68, 38.1603) -> (-75.5, 33.8301)
  line L375 (-75.5, 33.8301) -> (-75.5, 25.1699)
  line L376 (-51, 38.1603) -> (-58.5, 33.8301)
  line L377 (-43.5, 33.8301) -> (-51, 38.1603)
  line L378 (-43.5, 25.1699) -> (-43.5, 33.8301)
  line L379 (-51, 20.8397) -> (-43.5, 25.1699)
  line L380 (-42.5, 23.4378) -> (-50, 19.1077)
  line L381 (-50, 10.4474) -> (-42.5, 6.1173)
  line L382 (-35, 10.4474) -> (-35, 19.1077)
  line L383 (-35, 19.1077) -> (-42.5, 23.4378)
  line L384 (-8.5, 6.1173) -> (-1, 10.4474)
  line L385 (-16, 19.1077) -> (-16, 10.4474)
  line L386 (-18, 19.1077) -> (-25.5, 23.4378)
  line L387 (-26.5, 25.1699) -> (-26.5, 33.8301)
  line L388 (-34, 20.8397) -> (-26.5, 25.1699)
  line L389 (-25.5, 23.4378) -> (-33, 19.1077)
  line L390 (-18, 10.4474) -> (-18, 19.1077)
  line L391 (-25.5, 6.1173) -> (-18, 10.4474)
  line L392 (-33, 10.4474) -> (-25.5, 6.1173)
  line L393 (-33, 19.1077) -> (-33, 10.4474)
  line L394 (-41.5, 25.1699) -> (-34, 20.8397)
  line L395 (-24.5, 25.1699) -> (-17, 20.8397)
  line L396 (-24.5, 33.8301) -> (-24.5, 25.1699)
  line L397 (-26.5, 33.8301) -> (-34, 38.1603)
  line L398 (-34, 38.1603) -> (-41.5, 33.8301)
  line L399 (-41.5, 33.8301) -> (-41.5, 25.1699)
  line L400 (-17, 38.1603) -> (-24.5, 33.8301)
  line L401 (-9.5, 33.8301) -> (-17, 38.1603)
  line L402 (-9.5, 25.1699) -> (-9.5, 33.8301)
  line L403 (-17, 20.8397) -> (-9.5, 25.1699)
  line L404 (-8.5, 23.4378) -> (-16, 19.1077)
  line L405 (-16, 10.4474) -> (-8.5, 6.1173)
  line L406 (-1, 10.4474) -> (-1, 19.1077)
  line L407 (-1, 19.1077) -> (-8.5, 23.4378)
  line L408 (25.5, 6.1173) -> (33, 10.4474)
  line L409 (18, 19.1077) -> (18, 10.4474)
  line L410 (16, 19.1077) -> (8.5, 23.4378)
  line L411 (7.5, 25.1699) -> (7.5, 33.8301)
  line L412 (0, 20.8397) -> (7.5, 25.1699)
  line L413 (8.5, 23.4378) -> (1, 19.1077)
  line L414 (16, 10.4474) -> (16, 19.1077)
  line L415 (8.5, 6.1173) -> (16, 10.4474)
  line L416 (1, 10.4474) -> (8.5, 6.1173)
  line L417 (1, 19.1077) -> (1, 10.4474)
  line L418 (-7.5, 25.1699) -> (0, 20.8397)
  line L419 (9.5, 25.1699) -> (17, 20.8397)
  line L420 (9.5, 33.8301) -> (9.5, 25.1699)
  line L421 (7.5, 33.8301) -> (0, 38.1603)
  line L422 (0, 38.1603) -> (-7.5, 33.8301)
  line L423 (-7.5, 33.8301) -> (-7.5, 25.1699)
  line L424 (17, 38.1603) -> (9.5, 33.8301)
  line L425 (24.5, 33.8301) -> (17, 38.1603)
  line L426 (24.5, 25.1699) -> (24.5, 33.8301)
  line L427 (17, 20.8397) -> (24.5, 25.1699)
  line L428 (25.5, 23.4378) -> (18, 19.1077)
  line L429 (18, 10.4474) -> (25.5, 6.1173)
  line L430 (33, 10.4474) -> (33, 19.1077)
  line L431 (33, 19.1077) -> (25.5, 23.4378)
  line L432 (59.5, 6.1173) -> (67, 10.4474)
  line L433 (52, 19.1077) -> (52, 10.4474)
  line L434 (50, 19.1077) -> (42.5, 23.4378)
  line L435 (41.5, 25.1699) -> (41.5, 33.8301)
  line L436 (34, 20.8397) -> (41.5, 25.1699)
  line L437 (42.5, 23.4378) -> (35, 19.1077)
  line L438 (50, 10.4474) -> (50, 19.1077)
  line L439 (42.5, 6.1173) -> (50, 10.4474)
  line L440 (35, 10.4474) -> (42.5, 6.1173)
  line L441 (35, 19.1077) -> (35, 10.4474)
  line L442 (26.5, 25.1699) -> (34, 20.8397)
  line L443 (43.5, 25.1699) -> (51, 20.8397)
  line L444 (43.5, 33.8301) -> (43.5, 25.1699)
  line L445 (41.5, 33.8301) -> (34, 38.1603)
  line L446 (34, 38.1603) -> (26.5, 33.8301)
  line L447 (26.5, 33.8301) -> (26.5, 25.1699)
  line L448 (51, 38.1603) -> (43.5, 33.8301)
  line L449 (58.5, 33.8301) -> (51, 38.1603)
  line L450 (58.5, 25.1699) -> (58.5, 33.8301)
  line L451 (51, 20.8397) -> (58.5, 25.1699)
  line L452 (59.5, 23.4378) -> (52, 19.1077)
  line L453 (52, 10.4474) -> (59.5, 6.1173)
  line L454 (67, 10.4474) -> (67, 19.1077)
  line L455 (67, 19.1077) -> (59.5, 23.4378)
  line L456 (93.5, 6.1173) -> (101, 10.4474)
  line L457 (86, 19.1077) -> (86, 10.4474)
  line L458 (84, 19.1077) -> (76.5, 23.4378)
  line L459 (75.5, 25.1699) -> (75.5, 33.8301)
  line L460 (68, 20.8397) -> (75.5, 25.1699)
  line L461 (76.5, 23.4378) -> (69, 19.1077)
  line L462 (84, 10.4474) -> (84, 19.1077)
  line L463 (76.5, 6.1173) -> (84, 10.4474)
  line L464 (69, 10.4474) -> (76.5, 6.1173)
  line L465 (69, 19.1077) -> (69, 10.4474)
  line L466 (60.5, 25.1699) -> (68, 20.8397)
  line L467 (77.5, 25.1699) -> (85, 20.8397)
  line L468 (77.5, 33.8301) -> (77.5, 25.1699)
  line L469 (75.5, 33.8301) -> (68, 38.1603)
  line L470 (68, 38.1603) -> (60.5, 33.8301)
  line L471 (60.5, 33.8301) -> (60.5, 25.1699)
  line L472 (85, 38.1603) -> (77.5, 33.8301)
  line L473 (92.5, 33.8301) -> (85, 38.1603)
  line L474 (92.5, 25.1699) -> (92.5, 33.8301)
  line L475 (85, 20.8397) -> (92.5, 25.1699)
  line L476 (93.5, 23.4378) -> (86, 19.1077)
  line L477 (86, 10.4474) -> (93.5, 6.1173)
  line L478 (101, 10.4474) -> (101, 19.1077)
  line L479 (101, 19.1077) -> (93.5, 23.4378)
  line L480 (-42.5, 35.6173) -> (-35, 39.9474)
  line L481 (-50, 48.6077) -> (-50, 39.9474)
  line L482 (-52, 48.6077) -> (-59.5, 52.9378)
  line L483 (-60.5, 54.6699) -> (-60.5, 63.3301)
  line L484 (-68, 50.3397) -> (-60.5, 54.6699)
  line L485 (-59.5, 52.9378) -> (-67, 48.6077)
  line L486 (-52, 39.9474) -> (-52, 48.6077)
  line L487 (-59.5, 35.6173) -> (-52, 39.9474)
  line L488 (-67, 39.9474) -> (-59.5, 35.6173)
  line L489 (-67, 48.6077) -> (-67, 39.9474)
  line L490 (-75.5, 54.6699) -> (-68, 50.3397)
  line L491 (-58.5, 54.6699) -> (-51, 50.3397)
  line L492 (-58.5, 63.3301) -> (-58.5, 54.6699)
  line L493 (-60.5, 63.3301) -> (-68, 67.6603)
  line L494 (-68, 67.6603) -> (-75.5, 63.3301)
  line L495 (-75.5, 63.3301) -> (-75.5, 54.6699)
  line L496 (-51, 67.6603) -> (-58.5, 63.3301)
  line L497 (-43.5, 63.3301) -> (-51, 67.6603)
  line L498 (-43.5, 54.6699) -> (-43.5, 63.3301)
  line L499 (-51, 50.3397) -> (-43.5, 54.6699)
  line L500 (-42.5, 52.9378) -> (-50, 48.6077)
  line L501 (-50, 39.9474) -> (-42.5, 35.6173)
  line L502 (-35, 39.9474) -> (-35, 48.6077)
  line L503 (-35, 48.6077) -> (-42.5, 52.9378)
  line L504 (-8.5, 35.6173) -> (-1, 39.9474)
  line L505 (-16, 48.6077) -> (-16, 39.9474)
  line L506 (-18, 48.6077) -> (-25.5, 52.9378)
  line L507 (-26.5, 54.6699) -> (-26.5, 63.3301)
  line L508 (-34, 50.3397) -> (-26.5, 54.6699)
  line L509 (-25.5, 52.9378) -> (-33, 48.6077)
  line L510 (-18, 39.9474) -> (-18, 48.6077)
  line L511 (-25.5, 35.6173) -> (-18, 39.9474)
  line L512 (-33, 39.9474) -> (-25.5, 35.6173)
  line L513 (-33, 48.6077) -> (-33, 39.9474)
  line L514 (-41.5, 54.6699) -> (-34, 50.3397)
  line L515 (-24.5, 54.6699) -> (-17, 50.3397)
  line L516 (-24.5, 63.3301) -> (-24.5, 54.6699)
  line L517 (-26.5, 63.3301) -> (-34, 67.6603)
  line L518 (-34, 67.6603) -> (-41.5, 63.3301)
  line L519 (-41.5, 63.3301) -> (-41.5, 54.6699)
  line L520 (-17, 67.6603) -> (-24.5, 63.3301)
  line L521 (-9.5, 63.3301) -> (-17, 67.6603)
  line L522 (-9.5, 54.6699) -> (-9.5, 63.3301)
  line L523 (-17, 50.3397) -> (-9.5, 54.6699)
  line L524 (-8.5, 52.9378) -> (-16, 48.6077)
  line L525 (-16, 39.9474) -> (-8.5, 35.6173)
  line L526 (-1, 39.9474) -> (-1, 48.6077)
  line L527 (-1, 48.6077) -> (-8.5, 52.9378)
  line L528 (25.5, 35.6173) -> (33, 39.9474)
  line L529 (18, 48.6077) -> (18, 39.9474)
  line L530 (16, 48.6077) -> (8.5, 52.9378)
  line L531 (7.5, 54.6699) -> (7.5, 63.3301)
  line L532 (0, 50.3397) -> (7.5, 54.6699)
  line L533 (8.5, 52.9378) -> (1, 48.6077)
  line L534 (16, 39.9474) -> (16, 48.6077)
  line L535 (8.5, 35.6173) -> (16, 39.9474)
  line L536 (1, 39.9474) -> (8.5, 35.6173)
  line L537 (1, 48.6077) -> (1, 39.9474)
  line L538 (-7.5, 54.6699) -> (0, 50.3397)
  line L539 (9.5, 54.6699) -> (17, 50.3397)
  line L540 (9.5, 63.3301) -> (9.5, 54.6699)
  line L541 (7.5, 63.3301) -> (0, 67.6603)
  line L542 (0, 67.6603) -> (-7.5, 63.3301)
  line L543 (-7.5, 63.3301) -> (-7.5, 54.6699)
  line L544 (17, 67.6603) -> (9.5, 63.3301)
  line L545 (24.5, 63.3301) -> (17, 67.6603)
  line L546 (24.5, 54.6699) -> (24.5, 63.3301)
  line L547 (17, 50.3397) -> (24.5, 54.6699)
  line L548 (25.5, 52.9378) -> (18, 48.6077)
  line L549 (18, 39.9474) -> (25.5, 35.6173)
  line L550 (33, 39.9474) -> (33, 48.6077)
  line L551 (33, 48.6077) -> (25.5, 52.9378)
  line L552 (59.5, 35.6173) -> (67, 39.9474)
  line L553 (52, 48.6077) -> (52, 39.9474)
  line L554 (50, 48.6077) -> (42.5, 52.9378)
  line L555 (41.5, 54.6699) -> (41.5, 63.3301)
  line L556 (34, 50.3397) -> (41.5, 54.6699)
  line L557 (42.5, 52.9378) -> (35, 48.6077)
  line L558 (50, 39.9474) -> (50, 48.6077)
  line L559 (42.5, 35.6173) -> (50, 39.9474)
  line L560 (35, 39.9474) -> (42.5, 35.6173)
  line L561 (35, 48.6077) -> (35, 39.9474)
  line L562 (26.5, 54.6699) -> (34, 50.3397)
  line L563 (43.5, 54.6699) -> (51, 50.3397)
  line L564 (43.5, 63.3301) -> (43.5, 54.6699)
  line L565 (41.5, 63.3301) -> (34, 67.6603)
  line L566 (34, 67.6603) -> (26.5, 63.3301)
  line L567 (26.5, 63.3301) -> (26.5, 54.6699)
  line L568 (51, 67.6603) -> (43.5, 63.3301)
  line L569 (58.5, 63.3301) -> (51, 67.6603)
  line L570 (58.5, 54.6699) -> (58.5, 63.3301)
  line L571 (51, 50.3397) -> (58.5, 54.6699)
  line L572 (59.5, 52.9378) -> (52, 48.6077)
  line L573 (52, 39.9474) -> (59.5, 35.6173)
  line L574 (67, 39.9474) -> (67, 48.6077)
  line L575 (67, 48.6077) -> (59.5, 52.9378)
  line L576 (93.5, 35.6173) -> (101, 39.9474)
  line L577 (86, 48.6077) -> (86, 39.9474)
  line L578 (84, 48.6077) -> (76.5, 52.9378)
  line L579 (75.5, 54.6699) -> (75.5, 63.3301)
  line L580 (68, 50.3397) -> (75.5, 54.6699)
  line L581 (76.5, 52.9378) -> (69, 48.6077)
  line L582 (84, 39.9474) -> (84, 48.6077)
  line L583 (76.5, 35.6173) -> (84, 39.9474)
  line L584 (69, 39.9474) -> (76.5, 35.6173)
  line L585 (69, 48.6077) -> (69, 39.9474)
  line L586 (60.5, 54.6699) -> (68, 50.3397)
  line L587 (77.5, 54.6699) -> (85, 50.3397)
  line L588 (77.5, 63.3301) -> (77.5, 54.6699)
  line L589 (75.5, 63.3301) -> (68, 67.6603)
  line L590 (68, 67.6603) -> (60.5, 63.3301)
  line L591 (60.5, 63.3301) -> (60.5, 54.6699)
  line L592 (85, 67.6603) -> (77.5, 63.3301)
  line L593 (92.5, 63.3301) -> (85, 67.6603)
  line L594 (92.5, 54.6699) -> (92.5, 63.3301)
  line L595 (85, 50.3397) -> (92.5, 54.6699)
  line L596 (93.5, 52.9378) -> (86, 48.6077)
  line L597 (86, 39.9474) -> (93.5, 35.6173)
  line L598 (101, 39.9474) -> (101, 48.6077)
  line L599 (101, 48.6077) -> (93.5, 52.9378)
  line L600 (-40.5, -41.5) -> (40.5, -41.5)
  line L601 (40.5, -41.5) -> (40.5, 41.5)
  line L602 (40.5, 41.5) -> (-40.5, 41.5)
  line L603 (-40.5, 41.5) -> (-40.5, -41.5)
  line L604 (-40.5, -41.5) -> (40.5, 41.5) construction
  line L605 (40.5, -41.5) -> (-40.5, 41.5) construction
  point P0 (17, 0)
  point P1 (8.5, -14.7224)
  point P2 (25.5, -14.7224)
  point P3 (-59.5, -73.7224)
  point P4 (-25.5, -73.7224)
  point P5 (8.5, -73.7224)
  point P6 (42.5, -73.7224)
  point P7 (76.5, -73.7224)
  point P8 (-59.5, -44.2224)
  point P9 (-25.5, -44.2224)
  point P10 (8.5, -44.2224)
  point P11 (42.5, -44.2224)
  point P12 (76.5, -44.2224)
  point P13 (-59.5, -14.7224)
  point P14 (-25.5, -14.7224)
  point P15 (42.5, -14.7224)
  point P16 (76.5, -14.7224)
  point P17 (-59.5, 14.7776)
  point P18 (-25.5, 14.7776)
  point P19 (8.5, 14.7776)
  point P20 (42.5, 14.7776)
  point P21 (76.5, 14.7776)
  point P22 (-59.5, 44.2776)
  point P23 (-25.5, 44.2776)
  point P24 (8.5, 44.2776)
  point P25 (42.5, 44.2776)
  point P26 (76.5, 44.2776)
  point P27 (-40.5, -41.5)
  dimension "d81" = 7.5
  dimension "d82" = 7.5
  dimension "d83" = 2
  dimension "d84" = 7.5
  dimension "d85" = 2
  dimension "d86" = 2
  dimension "d87" = 7.5
  dimension "d88" = 2
  dimension "d89" = 2
  dimension "d92" = 68
  dimension "d93" = 59
  constraint horizontal L600
  constraint perpendicular L600 L601
  constraint parallel L600 L602
  constraint parallel L601 L603
  constraint coincident P27 L600.start
  constraint coincident L604 origin
  constraint coincident L605 origin
  measures "d81" distance of origin L5
  measures "d82" distance of P0 L11
  measures "d83" distance of L2 L11
  measures "d84" distance of P1 L17
  measures "d85" distance of L1 L16
  measures "d86" distance of L6 L15
  measures "d87" distance of P2 L23
  measures "d88" distance of L14 L23
  measures "d89" distance of L7 L22
extrude "Extrude12" add sketch "Sketch17" against normal blind 3 contours L166 L167 L169 L170 L171 L172 L173 L174 L177 L178 L181 L182 L188 L190 L191 L193 L194 L197 L198 L201 L212 L214 L215 L220 L221 L225 L226 L229 L230 L231 L264 L286 L287 L291 L292 L298 L301 L302 L316 L317 L320 L321 L322 L325 L326 L327 L360 L382 L383 L387 L388 L394 L397 L398 L436 L437 L440 L441 L442 L445 L446 L447 L480 L502 L504 L505 L510 L511 L512 L513 L525 L526 L528 L529 L534 L535 L536 L537 L549 L550 L560 L561 L600 L601 L602 L603
sketch "Sketch18" plane through (0, 3, 0) normal (0, 1, 0) x (-1, 0, 0)
  line L0 (-35.75, 34.75) -> (35.75, 34.75) construction
  line L1 (35.75, 34.75) -> (35.75, -36.75) construction
  line L2 (35.75, -36.75) -> (-35.75, -36.75) construction
  line L3 (-35.75, -36.75) -> (-35.75, 34.75) construction
  line L4 (-35.75, 34.75) -> (35.75, -36.75) construction
  line L5 (35.75, 34.75) -> (-35.75, -36.75) construction
  line L6 (40.5, -41.5) -> (-40.5, 39.5) construction
  point P0 (0, -1)
  dimension "d98" = 71.5
  dimension "d99" = 71.5
  constraint horizontal L0
  constraint perpendicular L0 L1
  constraint parallel L0 L2
  constraint parallel L1 L3
  constraint coincident L4 P0
  constraint coincident L5 P0
  constraint midpoint P0 L6
  measures "d98" distance of L1.end L2.end
  measures "d99" distance of L0.end L1.end
hole "Hole4" at (-35.75, 3, -36.75) at (35.75, 3, -36.75) at (-35.75, 3, 34.75) at (35.75, 3, 34.75) direction (0, -1, 0) diameter 4.5 end through all
